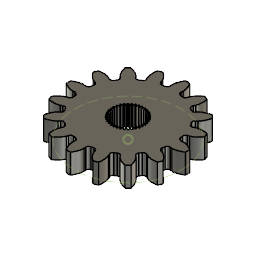
PIÑON_SERVO (Autodesk Fusion 360 design; units mm, degrees)
description: Spur Gear; Module: 1.0; Num Teeth: 16; Pressure Angle: 20.0; Backlash: 0.00 mm
Autodesk Fusion 360 part; units mm, degrees
sketch "Boceto1" plane through (0, 0, 0) normal (0, 0, 1) x (1, 0, 0)
  circle A0 centre (0, 0) radius 1.2447
  line L0 (2.0251, -1.3152) -> (1.7533, -0.9959)
  line L1 (1.0204, -1.7391) -> (1.3435, -2.0064)
  arc A1 (2.1667, -1.0658) -> (2.2227, -0.9436) centre (0, 0) ccw
  line L2 (1.5537, -1.2852) -> (1.9487, -1.4258)
  arc A2 (2.3189, -0.6734) -> (2.3528, -0.5433) centre (0, 0) ccw
  arc A3 (0.9747, -2.2092) -> (1.0961, -2.1515) centre (0, 0) ccw
  line L3 (1.8996, -0.6763) -> (2.3189, -0.6734)
  line L4 (0.7059, -2.3092) -> (0.7029, -1.8899)
  line L5 (0.7029, -1.8899) -> (0.9747, -2.2092)
  line L6 (-0.1265, -2.4113) -> (0.0142, -2.0163)
  arc A4 (1.9487, -1.4258) -> (2.0251, -1.3152) centre (0, 0) ccw
  arc A5 (1.3435, -2.0064) -> (1.4531, -1.9285) centre (0, 0) ccw
  arc A6 (-0.2605, -2.4006) -> (-0.1265, -2.4113) centre (0, 0) ccw
  line L7 (2.3528, -0.5433) -> (1.9881, -0.3362)
  line L8 (1.4531, -1.9285) -> (1.3069, -1.5355)
  line L9 (1.7533, -0.9959) -> (2.1667, -1.0658)
  circle A7 centre (0, 0) radius 0.7966
  line L10 (-0.3362, -1.9881) -> (-0.2605, -2.4006)
  line L11 (1.0961, -2.1515) -> (1.0204, -1.7391)
  line L12 (0.3641, -1.9832) -> (0.5763, -2.3449)
  arc A8 (0.1604, -2.4093) -> (0.2942, -2.3967) centre (0, 0) ccw
  line L13 (1.7659, -1.6469) -> (1.5537, -1.2852)
  line L14 (1.3069, -1.5355) -> (1.6715, -1.7426)
  line L15 (2.2227, -0.9436) -> (1.8996, -0.6763)
  line L16 (0.0142, -2.0163) -> (0.1604, -2.4093)
  arc A9 (0.5763, -2.3449) -> (0.7059, -2.3092) centre (0, 0) ccw
  line L17 (0.2942, -2.3967) -> (0.3641, -1.9832)
  arc A10 (1.6715, -1.7426) -> (1.7659, -1.6469) centre (0, 0) ccw
  arc A11 (1.4258, 1.9487) -> (1.3152, 2.0251) centre (0, 0) ccw
  line L18 (1.9285, 1.4531) -> (1.5355, 1.3069)
  arc A12 (-2.0064, -1.3435) -> (-1.9285, -1.4531) centre (0, 0) ccw
  line L19 (-0.9436, -2.2227) -> (-0.6763, -1.8996)
  arc A13 (0.6734, 2.3189) -> (0.5433, 2.3528) centre (0, 0) ccw
  line L20 (-1.9285, -1.4531) -> (-1.5355, -1.3069)
  line L21 (2.3092, 0.7059) -> (1.8899, 0.7029)
  line L22 (2.0163, 0.0142) -> (2.4093, 0.1604)
  line L23 (-2.3967, -0.2942) -> (-1.9832, -0.3641)
  arc A14 (1.0658, 2.1667) -> (0.9436, 2.2227) centre (0, 0) ccw
  line L24 (-1.0204, 1.7391) -> (-1.3435, 2.0064)
  line L25 (-2.4113, 0.1265) -> (-2.0163, -0.0142)
  line L26 (0.6763, 1.8996) -> (0.6734, 2.3189)
  arc A15 (2.2092, 0.9747) -> (2.1515, 1.0961) centre (0, 0) ccw
  line L27 (1.6469, 1.7659) -> (1.2852, 1.5537)
  line L28 (-0.6763, -1.8996) -> (-0.6734, -2.3189)
  arc A16 (-1.4258, -1.9487) -> (-1.3152, -2.0251) centre (0, 0) ccw
  arc A17 (-2.2092, -0.9747) -> (-2.1515, -1.0961) centre (0, 0) ccw
  line L29 (-1.9881, 0.3362) -> (-2.4006, 0.2605)
  line L30 (1.5355, 1.3069) -> (1.7426, 1.6715)
  line L31 (-1.5355, -1.3069) -> (-1.7426, -1.6715)
  line L32 (2.1515, 1.0961) -> (1.7391, 1.0204)
  line L33 (-1.8899, -0.7029) -> (-2.2092, -0.9747)
  line L34 (-0.5433, -2.3528) -> (-0.3362, -1.9881)
  line L35 (2.4113, -0.1265) -> (2.0163, 0.0142)
  line L36 (-1.9832, -0.3641) -> (-2.3449, -0.5763)
  arc A18 (2.4006, -0.2605) -> (2.4113, -0.1265) centre (0, 0) ccw
  arc A19 (-1.3435, 2.0064) -> (-1.4531, 1.9285) centre (0, 0) ccw
  line L37 (2.3967, 0.2942) -> (1.9832, 0.3641)
  arc A20 (-2.4093, -0.1604) -> (-2.3967, -0.2942) centre (0, 0) ccw
  line L38 (-0.7059, 2.3092) -> (-0.7029, 1.8899)
  line L39 (0.5433, 2.3528) -> (0.3362, 1.9881)
  line L40 (1.2852, 1.5537) -> (1.4258, 1.9487)
  arc A21 (-0.6734, -2.3189) -> (-0.5433, -2.3528) centre (0, 0) ccw
  line L41 (1.8899, 0.7029) -> (2.2092, 0.9747)
  line L42 (-0.7029, 1.8899) -> (-0.9747, 2.2092)
  line L43 (-2.3092, -0.7059) -> (-1.8899, -0.7029)
  arc A22 (-2.3449, -0.5763) -> (-2.3092, -0.7059) centre (0, 0) ccw
  line L44 (-0.0142, 2.0163) -> (-0.1604, 2.4093)
  line L45 (-2.1515, -1.0961) -> (-1.7391, -1.0204)
  line L46 (1.3152, 2.0251) -> (0.9959, 1.7533)
  line L47 (-1.5537, 1.2852) -> (-1.9487, 1.4258)
  arc A23 (2.3449, 0.5763) -> (2.3092, 0.7059) centre (0, 0) ccw
  line L48 (-0.3641, 1.9832) -> (-0.5763, 2.3449)
  line L49 (0.9436, 2.2227) -> (0.6763, 1.8996)
  line L50 (-2.0163, -0.0142) -> (-2.4093, -0.1604)
  line L51 (-1.7659, 1.6469) -> (-1.5537, 1.2852)
  line L52 (0.3362, 1.9881) -> (0.2605, 2.4006)
  arc A24 (-0.5763, 2.3449) -> (-0.7059, 2.3092) centre (0, 0) ccw
  arc A25 (-2.3189, 0.6734) -> (-2.3528, 0.5433) centre (0, 0) ccw
  arc A26 (-1.0658, -2.1667) -> (-0.9436, -2.2227) centre (0, 0) ccw
  line L53 (-1.2852, -1.5537) -> (-1.4258, -1.9487)
  arc A27 (-1.6715, 1.7426) -> (-1.7659, 1.6469) centre (0, 0) ccw
  line L54 (1.7391, 1.0204) -> (2.0064, 1.3435)
  arc A28 (-2.4006, 0.2605) -> (-2.4113, 0.1265) centre (0, 0) ccw
  line L55 (-2.2227, 0.9436) -> (-1.8996, 0.6763)
  arc A29 (-2.1667, 1.0658) -> (-2.2227, 0.9436) centre (0, 0) ccw
  line L56 (-0.9959, -1.7533) -> (-1.0658, -2.1667)
  arc A30 (2.4093, 0.1604) -> (2.3967, 0.2942) centre (0, 0) ccw
  arc A31 (2.0064, 1.3435) -> (1.9285, 1.4531) centre (0, 0) ccw
  arc A32 (-0.1604, 2.4093) -> (-0.2942, 2.3967) centre (0, 0) ccw
  line L57 (-1.3152, -2.0251) -> (-0.9959, -1.7533)
  arc A33 (-0.9747, 2.2092) -> (-1.0961, 2.1515) centre (0, 0) ccw
  line L58 (0.9959, 1.7533) -> (1.0658, 2.1667)
  arc A34 (-1.9487, 1.4258) -> (-2.0251, 1.3152) centre (0, 0) ccw
  arc A35 (-1.7426, -1.6715) -> (-1.6469, -1.7659) centre (0, 0) ccw
  line L59 (1.9832, 0.3641) -> (2.3449, 0.5763)
  line L60 (1.9881, -0.3362) -> (2.4006, -0.2605)
  line L61 (-1.8996, 0.6763) -> (-2.3189, 0.6734)
  line L62 (-0.2942, 2.3967) -> (-0.3641, 1.9832)
  line L63 (-1.7533, 0.9959) -> (-2.1667, 1.0658)
  line L64 (-1.6469, -1.7659) -> (-1.2852, -1.5537)
  line L65 (-1.7391, -1.0204) -> (-2.0064, -1.3435)
  arc A36 (1.7426, 1.6715) -> (1.6469, 1.7659) centre (0, 0) ccw
  line L66 (-1.3069, 1.5355) -> (-1.6715, 1.7426)
  line L67 (-2.3528, 0.5433) -> (-1.9881, 0.3362)
  line L68 (0.1265, 2.4113) -> (-0.0142, 2.0163)
  line L69 (-2.0251, 1.3152) -> (-1.7533, 0.9959)
  line L70 (-1.4531, 1.9285) -> (-1.3069, 1.5355)
  arc A37 (0.2605, 2.4006) -> (0.1265, 2.4113) centre (0, 0) ccw
  line L71 (-1.0961, 2.1515) -> (-1.0204, 1.7391)
  constraint coincident A0.centre A1.centre
pattern_circular "Patrón C1" [no effect]
extrude "Extruir4" cut sketch "Boceto1" along normal blind 8 contours A0
sketch "Boceto5" plane through (0, 0, 0) normal (0, 0, 1) x (1, 0, 0)
  circle A0 centre (0, 0) radius 6.843
  circle A1 centre (0, 0) radius 1
extrude "Extruir5" add sketch "Boceto5" along normal blind 3 separate body
sketch "Boceto6" plane through (0, 0, 0) normal (0, 0, 1) x (1, 0, 0)
  spline S0 degree 5 poles (7.4695, -0.8483) (7.4738, -0.8488) (7.4825, -0.8496) (7.4954, -0.8505) (7.5128, -0.851) (7.5345, -0.8507) (7.5562, -0.8497) (7.578, -0.8483) (7.5999, -0.8466) (7.6217, -0.8447) (7.6436, -0.8427) (7.6654, -0.8405) (7.6873, -0.838) (7.7092, -0.8351) (7.7312, -0.8319) (7.7531, -0.8284) (7.775, -0.8246) (7.797, -0.8206) (7.819, -0.8164) (7.8409, -0.812) (7.8629, -0.8074) (7.8849, -0.8026) (7.9068, -0.7976) (7.9288, -0.7924) (7.9508, -0.7869) (7.9728, -0.7813) (7.9947, -0.7754) (8.0167, -0.7694) (8.0387, -0.7632) (8.0607, -0.7568) (8.0826, -0.7503) (8.1046, -0.7435) (8.1265, -0.7366) (8.1485, -0.7295) (8.1704, -0.7222) (8.1924, -0.7148) (8.2143, -0.7072) (8.2362, -0.6994) (8.2581, -0.6915) (8.28, -0.6834) (8.3019, -0.6751) (8.3238, -0.6667) (8.3457, -0.6581) (8.3675, -0.6494) (8.3894, -0.6405) (8.4112, -0.6315) (8.433, -0.6223) (8.4548, -0.6129) (8.4766, -0.6034) (8.4984, -0.5938) (8.5202, -0.584) (8.5419, -0.574) (8.5636, -0.564) (8.5853, -0.5537) (8.607, -0.5433) (8.6287, -0.5328) (8.6503, -0.5222) (8.672, -0.5113) (8.6936, -0.5004) (8.7152, -0.4893) (8.7368, -0.4781) (8.7583, -0.4667) (8.7798, -0.4552) (8.8013, -0.4436) (8.8228, -0.4318) (8.8443, -0.4199) (8.8657, -0.4079) (8.8872, -0.3957) (8.9085, -0.3834) (8.9299, -0.3709) (8.9512, -0.3584) (8.9683, -0.3482) (8.9811, -0.3405) (8.9896, -0.3354) (8.9938, -0.3328) knots 0 0 0 0 0 0 0.01428571 0.02857143 0.04285714 0.05714286 0.07142857 0.08571429 0.1 0.11428571 0.12857143 0.14285714 0.15714286 0.17142857 0.18571429 0.2 0.21428571 0.22857143 0.24285714 0.25714286 0.27142857 0.28571429 0.3 0.31428571 0.32857143 0.34285714 0.35714286 0.37142857 0.38571429 0.4 0.41428571 0.42857143 0.44285714 0.45714286 0.47142857 0.48571429 0.5 0.51428571 0.52857143 0.54285714 0.55714286 0.57142857 0.58571429 0.6 0.61428571 0.62857143 0.64285714 0.65714286 0.67142857 0.68571429 0.7 0.71428571 0.72857143 0.74285714 0.75714286 0.77142857 0.78571429 0.8 0.81428571 0.82857143 0.84285714 0.85714286 0.87142857 0.88571429 0.9 0.91428571 0.92857143 0.94285714 0.95714286 0.97142857 0.98571429 1 1 1 1 1 1
  spline S1 degree 5 poles (7.4695, 0.8483) (7.4738, 0.8488) (7.4825, 0.8496) (7.4954, 0.8505) (7.5128, 0.851) (7.5345, 0.8507) (7.5562, 0.8497) (7.578, 0.8483) (7.5999, 0.8466) (7.6217, 0.8447) (7.6436, 0.8427) (7.6654, 0.8405) (7.6873, 0.838) (7.7092, 0.8351) (7.7312, 0.8319) (7.7531, 0.8284) (7.775, 0.8246) (7.797, 0.8206) (7.819, 0.8164) (7.8409, 0.812) (7.8629, 0.8074) (7.8849, 0.8026) (7.9068, 0.7976) (7.9288, 0.7924) (7.9508, 0.7869) (7.9728, 0.7813) (7.9947, 0.7754) (8.0167, 0.7694) (8.0387, 0.7632) (8.0607, 0.7568) (8.0826, 0.7503) (8.1046, 0.7435) (8.1265, 0.7366) (8.1485, 0.7295) (8.1704, 0.7222) (8.1924, 0.7148) (8.2143, 0.7072) (8.2362, 0.6994) (8.2581, 0.6915) (8.28, 0.6834) (8.3019, 0.6751) (8.3238, 0.6667) (8.3457, 0.6581) (8.3675, 0.6494) (8.3894, 0.6405) (8.4112, 0.6315) (8.433, 0.6223) (8.4548, 0.6129) (8.4766, 0.6034) (8.4984, 0.5938) (8.5202, 0.584) (8.5419, 0.574) (8.5636, 0.564) (8.5853, 0.5537) (8.607, 0.5433) (8.6287, 0.5328) (8.6503, 0.5222) (8.672, 0.5113) (8.6936, 0.5004) (8.7152, 0.4893) (8.7368, 0.4781) (8.7583, 0.4667) (8.7798, 0.4552) (8.8013, 0.4436) (8.8228, 0.4318) (8.8443, 0.4199) (8.8657, 0.4079) (8.8872, 0.3957) (8.9085, 0.3834) (8.9299, 0.3709) (8.9512, 0.3584) (8.9683, 0.3482) (8.9811, 0.3405) (8.9896, 0.3354) (8.9938, 0.3328) knots 0 0 0 0 0 0 0.01428571 0.02857143 0.04285714 0.05714286 0.07142857 0.08571429 0.1 0.11428571 0.12857143 0.14285714 0.15714286 0.17142857 0.18571429 0.2 0.21428571 0.22857143 0.24285714 0.25714286 0.27142857 0.28571429 0.3 0.31428571 0.32857143 0.34285714 0.35714286 0.37142857 0.38571429 0.4 0.41428571 0.42857143 0.44285714 0.45714286 0.47142857 0.48571429 0.5 0.51428571 0.52857143 0.54285714 0.55714286 0.57142857 0.58571429 0.6 0.61428571 0.62857143 0.64285714 0.65714286 0.67142857 0.68571429 0.7 0.71428571 0.72857143 0.74285714 0.75714286 0.77142857 0.78571429 0.8 0.81428571 0.82857143 0.84285714 0.85714286 0.87142857 0.88571429 0.9 0.91428571 0.92857143 0.94285714 0.95714286 0.97142857 0.98571429 1 1 1 1 1 1
  arc A0 (8.9938, -0.3328) -> (8.9938, 0.3328) centre (0, 0) ccw
  line L0 (6.7894, -0.771) -> (7.4695, -0.8483)
  line L1 (6.7894, 0.771) -> (7.4695, 0.8483)
  line L2 (6.7894, -0.771) -> (6.7894, 0.771)
  point P0 (7.5761, -0.8484)
  point P1 (7.6837, -0.8383)
  point P2 (7.792, -0.8215)
  point P3 (7.9008, -0.7989)
  point P4 (8.0099, -0.7712)
  point P5 (8.1193, -0.7388)
  point P6 (8.2289, -0.702)
  point P7 (8.3385, -0.6609)
  point P8 (8.4481, -0.6158)
  point P9 (8.5577, -0.5667)
  point P10 (8.6671, -0.5137)
  point P11 (8.7763, -0.4571)
  point P12 (8.8853, -0.3967)
  point P13 (7.5761, 0.8484)
  point P14 (7.6837, 0.8383)
  point P15 (7.792, 0.8215)
  point P16 (7.9008, 0.7989)
  point P17 (8.0099, 0.7712)
  point P18 (8.1193, 0.7388)
  point P19 (8.2289, 0.702)
  point P20 (8.3385, 0.6609)
  point P21 (8.4481, 0.6158)
  point P22 (8.5577, 0.5667)
  point P23 (8.6671, 0.5137)
  point P24 (8.7763, 0.4571)
  point P25 (8.8853, 0.3967)
extrude "Extruir6" add sketch "Boceto6" along normal blind 3
fillet "Empalme2" radius 0.4 2 edges at (6.7993, -0.7722, 1.5) (6.7993, 0.7722, 1.5)
pattern_circular "Patrón C2" count 16 over 360 about axis through (0, 0, 0) along (0, 0, 1) of "Extruir6", "Empalme2"
sketch "Boceto7" plane through (0, 0, 0) normal (0, 0, 1) x (1, 0, 0)
  circle A0 centre (0, 0) radius 8 construction
extrude "Extruir7" cut sketch "Boceto1" along normal blind 5 contours A0 | L0 L1 A1 L2 A2 A3 L3 L4 L5 L6 A4 A5 A6 L7 L8 L9 L10 L11 L12 A8 L13 L14 L15 L16 A9 L17 A10 A11 L18 A12 L19 A13 L20 L21 L22 L23 A14 L24 L25 L26 A15 L27 L28 A16 A17 L29 L30 L31 L32 L33 L34 L35 L36 A18 A19 L37 A20 L38 L39 L40 A21 L41 L42 L43 A22 L44 L45 L46 L47 A23 L48 L49 L50 L51 L52 A24 A25 A26 L53 A27 L54 A28 L55 A29 L56 A30 A31 A32 L57 A33 L58 A34 A35 L59 L60 L61 L62 L63 L64 L65 A36 L66 L67 L68 L69 L70 A37 L71
named bodies: "Spur Gear (16 teeth)"
